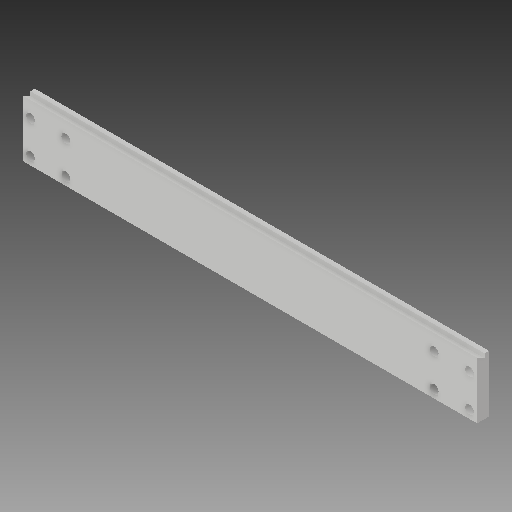
# Autodesk Inventor part: SuportePincas
Saved by Autodesk Inventor 2018 (Build 220112000, 112)
## iProperties
Created: 2018-07-24
Part Number: SuportePincas
Material: Genérico
Document SubType Name: Modeling
Designer: Usuario
Density: 1 g/cm^3
Appearance: Padrão
Mass: 148.202 g
Surface Area: 427.583 cm^2
Volume: 148.202 cm^3
Author: Usuario
Autodesk Inventor part; units mm, degrees
ref_plane "YZ Plane" through (0, 0, 0) normal (1, 0, 0) x (0, 1, 0)
ref_plane "XZ Plane" through (0, 0, 0) normal (0, 1, 0) x (-1, 0, 0)
ref_plane "XY Plane" through (0, 0, 0) normal (0, 0, 1) x (1, 0, 0)
sketch "Esboço1" plane through (0, 0, 0) normal (0, 0, 1) x (1, 0, 0)
  line L0 (30.4895, -39) -> (-329.5105, -39)
  line L1 (-329.5105, -39) -> (-329.5105, 6)
  line L2 (-329.5105, 6) -> (30.4895, 6)
  line L3 (30.4895, 6) -> (30.4895, -39)
  point P0 (0, 0)
  point P1 (-329.5105, 0)
  dimension "d0" = 45
  constraints: 8 end point, 2 horizontal, 2 parallel, 1 perpendicular
  measures "d0" distance of L0.end L1.end
extrude "Extrusão1" add sketch "Esboço1" along normal blind 9.52
sketch "Esboço2" plane through (0, 0, 9.52) normal (0, 0, 1) x (1, 0, 0)
  circle A0 centre (24.4895, -32.5) radius 2.067 projected
  circle A1 centre (24.4895, -6.5) radius 2.067 projected
  circle A2 centre (-3.5105, -6.5) radius 2.067 projected
  circle A3 centre (-3.5105, -32.5) radius 2.067 projected
  circle A4 centre (-323.5105, -32.5) radius 2.067 projected
  circle A5 centre (-295.5105, -32.5) radius 2.067 projected
  circle A6 centre (-295.5105, -6.5) radius 2.067 projected
  circle A7 centre (-323.5105, -6.5) radius 2.067 projected
  point P0 (0, 0)
hole "Furo1" at (24.4895, -32.5, 9.52) at (-3.5105, -32.5, 9.52) at (-3.5105, -6.5, 9.52) at (24.4895, -6.5, 9.52) at (-323.5105, -32.5, 9.52) at (-295.5105, -32.5, 9.52) at (-295.5105, -6.5, 9.52) at (-323.5105, -6.5, 9.52) direction (0, 0, -1) diameter 5.5 end through all counterbore diameter 7 counterbore depth 4
sketch "Esboço3" plane through (30.4895, -39, 0) normal (1, 0, 0) x (0, 0, -1)
  line L0 (0, 45) -> (-9.52, 45) projected
  line L1 (-9.52, 45) -> (-3.52, 41.5359)
  line L2 (-9.52, 45) -> (-2.5918, 45) construction
  line L3 (-3.52, 41.5359) -> (-3.52, 45)
  point P0 (0, 39)
  dimension "d10" = 30
  dimension "d13" = 6
  constraints: 6 end point, 1 equal length, 1 horizontal, 1 point on line, 1 vertical
  measures "d10" angle of L1 L2
  measures "d13" distance of L3.end L0.end
extrude "Extrusão2" cut sketch "Esboço3" against normal through all
